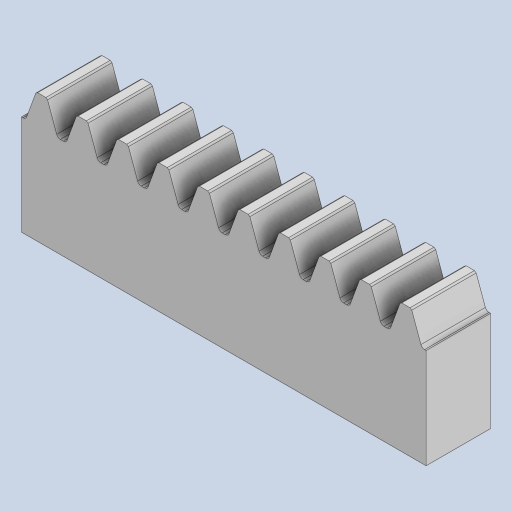
# Autodesk Inventor part: tume
Saved by Autodesk Inventor 2023 (Build 270158000, 158)
## iProperties
Created: 2024-11-27
Part Number: tume
Material: Generic
Document SubType Name: Modeling
Designer: kiyo
Density: 1 g/cm^3
Appearance: Default
Author: kiyo
Autodesk Inventor part; units mm, degrees
ref_plane "YZ Plane" through (0, 0, 0) normal (1, 0, 0) x (0, 1, 0)
ref_plane "XZ Plane" through (0, 0, 0) normal (0, 1, 0) x (-1, 0, 0)
ref_plane "XY Plane" through (0, 0, 0) normal (0, 0, 1) x (1, 0, 0)
sketch "スケッチ3" plane through (0, 0, 0) normal (0, 1, 0) x (-1, 0, 0)
  line L0 (0, 0) -> (5, 0)
  line L1 (5, 0) -> (5, 10)
  line L2 (5, 10) -> (0, 10)
  line L3 (0, 10) -> (0, 0)
  line L4 (0, 6) -> (-4, 6)
  line L5 (-4, 6) -> (-4, 4)
  line L6 (-4, 4) -> (0, 4)
  line L7 (0, 4) -> (0, 6)
  line L8 (-4, 25) -> (-39, 25)
  line L9 (-39, 25) -> (-39, -15)
  line L10 (-39, -15) -> (-4, -15)
  line L11 (-4, -15) -> (-4, 25)
  point P0 (0, 5)
  point P1 (0, 4)
  dimension "d5" = 5
  dimension "d6" = 10
  dimension "d7" = 4
  dimension "d8" = 2
  dimension "d9" = 35
  dimension "d10" = 4
  dimension "d11" = 40
  dimension "d12" = 20
  constraints: 24 end point, 6 parallel, 3 horizontal, 3 perpendicular, 2 point on line, 1 midpoint
  measures "d5" distance of L1.end L2.end
  measures "d6" distance of L0.end L1.end
  measures "d7" distance between parallel lines of L4 L2
  measures "d8" distance between parallel lines of L6 L4
  measures "d9" distance of L8.start L8.end
  measures "d10" distance of L5.end L6.end
  measures "d11" distance of L8.end L9.end
  measures "d12" distance from line of point (0, 5) L8
extrude "押し出し2" add sketch "スケッチ3" along normal blind 10 and the other way blind 30 contours L3 L2 L1 L0
extrude "押し出し3" [suppressed]
sketch "スケッチ4" plane through (-5, -30, 10) normal (-1, 0, 0) x (0, 0, 1)
  line L0 (0, 38.8506) -> (-2.25, 39.6696)
  line L1 (0, 0) -> (0, 40) projected
  line L2 (0, 38.0078) -> (-2.25, 37.1888)
  line L3 (-10, 40) -> (0, 40) projected
  line L4 (0, 38.4292) -> (-2.25, 38.4292)
  line L5 (0, 40) -> (-10, 40) projected
  line L6 (-1, 40) -> (-1, 36.8584)
  line L7 (-2.25, 40) -> (-2.25, 36.8584)
  line L8 (0, 36.8584) -> (-2.25, 36.8584)
  line L9 (-1, 40) -> (-1, 39.2146)
  line L10 (-1, 39.2146) -> (-1, 38.4292)
  line L11 (-1, 38.4292) -> (-1, 37.6438)
  line L12 (-1, 37.6438) -> (-1, 36.8584)
  point P0 (-10, 30)
  dimension "d21" = 20
  dimension "d23" = 1
  dimension "d24" = 1.25
  dimension "d25" = 1.5708
  dimension "d27" = 1.5708
  dimension "d28" = 20
  constraints: 21 end point, 12 point on line, 3 collinear, 2 midpoint, 2 vertical, 1 horizontal, 1 perpendicular
  measures "d21" angle of L4 L0
  measures "d23" distance between parallel lines of L6 L1
  measures "d24" distance between parallel lines of L7 L6
  measures "d25" distance between parallel lines of L4 L3
  measures "d27" distance between parallel lines of L8 L4
  measures "d28" angle of L4 L2
extrude "押し出し4" cut sketch "スケッチ4" against normal blind 5 contours L0 L6 L3 L1 | L0 L7 L3 L6 | L1 L8 L6 L2 | L6 L8 L7 L2
fillet "フィレット1" radius 0.3 2 edges at (-2.5, 9.6696, 7.75) (-2.5, 7.1888, 7.75)
chamfer "面取り1" distance 0.1 angle 45 2 edges at (-2.5, 8.8506, 10) (-2.5, 8.0078, 10)
pattern_linear "矩形状パターン1" count 10 spacing 3.1416 along (0, -1, 0) of "押し出し4", "フィレット1", "面取り1"
sketch "スケッチ5" plane through (-5, -30, 0) normal (-1, 0, 0) x (0, 0, 1)
  line L0 (10, 8.5841) -> (10, 0) projected
  line L1 (10, 8.5841) -> (0, 8.5841)
  line L2 (0, 8.5841) -> (0, 0)
  line L3 (0, 0) -> (10, 0)
  line L4 (10, 0) -> (10, 8.5841)
  point P0 (0, 30)
  constraints: 8 end point, 2 parallel, 1 horizontal, 1 perpendicular
extrude "押し出し5" cut sketch "スケッチ5" against normal blind 10
equation "\"d12\" = 0.5 * d11"
equation "\"d23\" = module"
equation "\"d24\" = 1.25 * module"
equation "\"d25\" = 1.5708 * module"
equation "\"d27\" = d25"
equation "\"d28\" = d21"
equation "\"d37\" = 3.14159 * module"
equation "\"module\" = 1"
